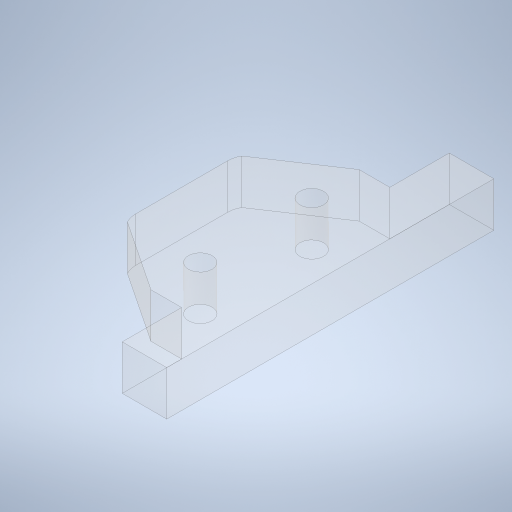
# Autodesk Inventor part: 射出_ベルト固定
Saved by Autodesk Inventor 2023 (Build 270158000, 158)
## iProperties
Created: 2022-04-23
Part Number: 射出_ベルト固定
Material: PET プラスチック
Document SubType Name: Modeling
Designer: yuta
Density: 1.541 g/cm^3
Appearance: ポリカーボネート - クリア
Author: yuta
Autodesk Inventor part; units mm, degrees
ref_plane "YZ Plane" through (0, 0, 0) normal (1, 0, 0) x (0, 1, 0)
ref_plane "XZ Plane" through (0, 0, 0) normal (0, 1, 0) x (-1, 0, 0)
ref_plane "XY Plane" through (0, 0, 0) normal (0, 0, 1) x (1, 0, 0)
sketch "スケッチ1" plane through (0, 0, 0) normal (0, 1, 0) x (-1, 0, 0)
  line L0 (0, 0) -> (6, 0)
  line L1 (0, -44) -> (0, 0)
  line L2 (6, 0) -> (6, -8)
  line L3 (6, -44) -> (6, -36)
  line L4 (6, -36) -> (16, -36)
  line L5 (6, -8) -> (16, -8)
  line L6 (6, -44) -> (0, -44)
  line L7 (16, -8) -> (20, -15)
  line L8 (16, -36) -> (20, -29)
  line L9 (20, -15) -> (20, -29)
  point P0 (0, -22)
  point P1 (10, -14.5)
  point P2 (10, -29.5)
  dimension "d2" = 8
  dimension "d3" = 6
  dimension "d4" = 8
  dimension "d5" = 6
  dimension "d9" = 10
  dimension "d10" = 10
  dimension "d11" = 10
  constraints: 20 end point, 3 parallel, 2 horizontal, 2 vertical, 1 midpoint, 1 perpendicular
  measures "d2" distance of L0.end L2.end
  measures "d3" distance between parallel lines of L1 L2
  measures "d4" distance of L3.start L3.end
  measures "d5" distance between parallel lines of L1 L3
  measures "d9" distance from line of L2 L5.end
  measures "d10" distance from line of L3 L4.end
  measures "d11" distance from line of L1 point (10, -14.5)
extrude "押し出し1" add sketch "スケッチ1" along normal blind 6
sketch "スケッチ2" plane through (0, 6, 0) normal (0, 1, 0) x (1, 0, 0)
  line L0 (0, 0) -> (0, 44) projected
  line L1 (-16, 8) -> (-6, 8) projected
  line L2 (-6, 36) -> (-16, 36) projected
  point P0 (-10, 14.5)
  point P1 (-10, 29.5)
  dimension "d17" = 10
  dimension "d18" = 6.5
  dimension "d19" = 10
  dimension "d20" = 6.5
  measures "d17" distance from line of point (-10, 14.5) L0
  measures "d18" distance from line of L1 point (-10, 14.5)
  measures "d19" distance from line of point (-10, 29.5) L0
  measures "d20" distance from line of L2 point (-10, 29.5)
hole "穴1" at (-10, 6, -14.5) at (-10, 6, -29.5) direction (0, -1, 0) diameter 3.2 end through all
fillet "フィレット1" radius 3 2 edges at (-16, 3, -8) (-16, 3, -36)
fillet "フィレット2" radius 3 2 edges at (-20, 3, -29) (-20, 3, -15)
sketch "スケッチ3" plane through (0, 6, 0) normal (0, 1, 0) x (1, 0, 0)
  arc A0 (-20, 15.7967) -> (-19.6047, 14.3083) centre (-17, 15.7967) ccw projected
  line L0 (-19.6047, 14.3083) -> (-10.1295, 8)
  line L1 (-14.259, 8) -> (-6, 8) projected
  line L2 (-20, 28.2033) -> (-20, 15.7967) projected
  line L3 (-20, 22) -> (-17.294, 22)
  line L4 (-19.6047, 29.6917) -> (-10.1295, 36)
  line L5 (-10.1295, 8) -> (-16.3751, 6.1485)
  line L6 (-19.6047, 14.3083) -> (-16.8638, 9.5116) projected
  line L7 (-16.3751, 6.1485) -> (-19.6047, 14.3083)
  line L8 (-16.8638, 34.4884) -> (-19.6047, 29.6917) projected
  line L9 (-19.6047, 29.6917) -> (-16.8449, 39.8374)
  line L10 (-16.8449, 39.8374) -> (-10.1295, 36)
  point P0 (0, 0)
  constraints: 14 end point, 2 midpoint, 2 symmetric about line, 1 horizontal, 1 perpendicular
extrude "押し出し2" cut sketch "スケッチ3" against normal blind 10
